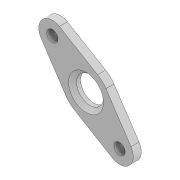
# Autodesk Inventor part: IM_Lensholder_macroscope
Saved by Autodesk Inventor 2022 (Build 260153000, 153)
## iProperties
Created: 2023-04-14
Part Number: IM_Lensholder_macroscope
Material: Generisch
Document SubType Name: Modeling
Designer: diederichbenedict
Density: 1 g/cm^3
Appearance: Vorgabe
Author: diederichbenedict
Autodesk Inventor part; units mm, degrees
ref_plane "YZ Plane" through (0, 0, 0) normal (1, 0, 0) x (0, 1, 0)
ref_plane "XZ Plane" through (0, 0, 0) normal (0, 1, 0) x (-1, 0, 0)
ref_plane "XY Plane" through (0, 0, 0) normal (0, 0, 1) x (1, 0, 0)
sketch "Skizze1" plane through (0, 0, 0) normal (0, 0, 1) x (1, 0, 0)
  circle A0 centre (0.0001, -0.0022) radius 3.9802 projected
  circle A1 centre (-8.37, 7.9978) radius 1.4 projected
  circle A2 centre (8.3745, -8.0022) radius 1.4 projected
  line L0 (-9.5383, 7.2264) -> (-3.2198, -2.3418)
  line L1 (-7.6522, 9.1998) -> (1.8915, 3.4999)
  line L2 (9.5428, -7.2307) -> (3.3215, 2.191)
  line L3 (-1.8517, -3.5253) -> (7.6567, -9.2041)
  point P0 (0, 0)
  constraints: 8 end point, 8 point on circle, 5 tangent, 1 parallel
extrude "Extrusion1" add sketch "Skizze1" along normal blind 2
sketch "Skizze2" plane through (0, 0, 2) normal (0, 0, 1) x (1, 0, 0)
  arc A0 (-7.6522, 9.1998) -> (-9.5383, 7.2264) centre (-8.37, 7.9978) ccw projected
  line L0 (-9.5383, 7.2264) -> (-3.2198, -2.3418) projected
  arc A1 (-3.2198, -2.3418) -> (-1.8517, -3.5253) centre (0.0001, -0.0022) ccw projected
  line L1 (-1.8517, -3.5253) -> (7.6567, -9.2041) projected
  arc A2 (7.6567, -9.2041) -> (9.5428, -7.2307) centre (8.3745, -8.0022) ccw projected
  line L2 (9.5428, -7.2307) -> (3.3215, 2.191) projected
  arc A3 (3.3215, 2.191) -> (1.8915, 3.4999) centre (0.0001, -0.0022) ccw projected
  line L3 (1.8915, 3.4999) -> (-7.6522, 9.1998) projected
  arc A4 (-6.6267, 10.9169) -> (-11.2072, 6.1243) centre (-8.37, 7.9978) ccw
  line L4 (-11.2072, 6.1243) -> (-4.8666, -3.4774)
  arc A5 (-4.8666, -3.4774) -> (-2.8352, -5.2674) centre (0.0001, -0.0022) ccw
  line L5 (-2.8352, -5.2674) -> (6.6312, -10.9212)
  arc A6 (6.6312, -10.9212) -> (11.2118, -6.1287) centre (8.3745, -8.0022) ccw
  line L6 (11.2118, -6.1287) -> (4.9905, 3.2931)
  arc A7 (4.9905, 3.2931) -> (2.8837, 5.2369) centre (0.0001, -0.0022) ccw
  line L7 (2.8837, 5.2369) -> (-6.6267, 10.9169)
  point P0 (0, 0)
  dimension "d2" = 2
  constraints: 8 end point, 8 point on circle, 4 centre point, 7 other
  measures "d2" distance between parallel lines of L3 L7
extrude "Extrusion2" add sketch "Skizze2" against normal up to surface (2 mm away)
sketch "Skizze3" plane through (0, 0, 2) normal (0, 0, 1) x (1, 0, 0)
  circle A0 centre (0.0001, -0.0022) radius 3.9802 projected
  circle A1 centre (-8.37, 7.9978) radius 1.4 projected
  circle A2 centre (8.3745, -8.0022) radius 1.4 projected
  circle A3 centre (0.0001, -0.0022) radius 3.35
  point P0 (0, 0)
  dimension "d5" = 6.7
  constraints: 1 centre point, 1 coincident
  measures "d5" diameter of A3
extrude "Extrusion3" cut sketch "Skizze3" against normal through all contours A1 | A2 | A3
sketch "Skizze4" plane through (0, 0, 2) normal (0, 0, 1) x (1, 0, 0)
  circle A0 centre (-8.37, 7.9978) radius 1.4 projected
  circle A1 centre (8.3745, -8.0022) radius 1.4 projected
  point P0 (0, 0)
hole "Bohrung1" at (-8.37, 7.9978, 2) at (8.3745, -8.0022, 2) direction (0, 0, -1) diameter 2.8 end through all
chamfer "Fase1" distance 1 angle 45 1 edges at (-3.3499, -0.0022, 2)
